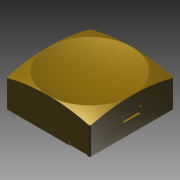
# Autodesk Inventor part: UB216SKG035D-1JBle_cap
Saved by Autodesk Inventor 2015 SP1 (Build 190203100, 203)
## iProperties
Category: Electrical
Company: Autodesk Inc.
Created: 2014-12-15
Part Number: UB216SKG035D-1JBle_cap
Catalog Web Link: http://www.nkkswitches.com/
Description: AT3074JB, AT3075B, AT3076JB-Illuminated Pushbuttons - Series UB2
Vendor: NKK Switches
Document SubType Name: Modeling
Designer: Autodesk Inc.
Manufacturer: NKKSWITCHES
Mass: 0.356668 g
Surface Area: 10.3147 cm^2
Volume: 0.356668 cm^3
Density: 1 g/cm^3
Material: Generic
Appearance: PSOLRGB-255-191-0
Title: UB216SKG035D-1JBle_cap
Author: Autodesk Inc.
Autodesk Inventor part; units mm, degrees
sketch "Sketch_2" plane through (0, 0, 0) normal (0, 0, 1) x (1, 0, 0)
  line L0 (-7.5057, 0.254) -> (7.5057, 0.254)
  line L1 (7.5057, 0.254) -> (7.5057, 6.096)
  line L2 (7.5057, 6.096) -> (-7.5057, 6.096)
  line L3 (-7.5057, 6.096) -> (-7.5057, 0.254)
  constraints: 8 end point
extrude "Extrusion1" add sketch "Sketch_2" along normal mid plane 15.0114
sketch "Sketch_20" plane through (0, 0, 0) normal (0, 1, 0) x (-1, 0, 0)
  line L0 (8.89, 8.89) -> (-8.89, 8.89)
  line L1 (-8.89, 8.89) -> (-8.89, -8.89)
  line L2 (-8.89, -8.89) -> (8.89, -8.89)
  line L3 (8.89, -8.89) -> (8.89, 8.89)
  line L4 (7.5057, -7.2517) -> (7.5057, 7.2517)
  arc A0 (7.5057, 7.2517) -> (7.2517, 7.5057) centre (7.2517, 7.2517) ccw
  line L5 (7.2517, 7.5057) -> (-7.2517, 7.5057)
  arc A1 (-7.2517, 7.5057) -> (-7.5057, 7.2517) centre (-7.2517, 7.2517) ccw
  line L6 (-7.5057, 7.2517) -> (-7.5057, -7.2517)
  arc A2 (-7.5057, -7.2517) -> (-7.2517, -7.5057) centre (-7.2517, -7.2517) ccw
  line L7 (-7.2517, -7.5057) -> (7.2517, -7.5057)
  arc A3 (7.2517, -7.5057) -> (7.5057, -7.2517) centre (7.2517, -7.2517) ccw
  constraints: 16 end point, 8 point on circle, 4 centre point
extrude "Extrusion2" cut sketch "Sketch_20" along normal blind 7.62
sketch "Sketch_9" plane through (0, 0, 0) normal (0.7071, 0, 0.7071) x (0.7071, 0, -0.7071)
  line L0 (0, 31.496) -> (0, 5.0196)
  arc A0 (-7.5057, 6.096) -> (0, 5.0196) centre (0, 31.7268) ccw
  arc A1 (-7.5057, 6.096) -> (-10.6172, 5.08) centre (0, -22.1627) ccw
  line L1 (-10.6172, 5.08) -> (-10.6172, 31.496)
  line L2 (-10.6172, 31.496) -> (0, 31.496)
  line L3 (0, 31.496) -> (0, 5.0196)
  constraints: 8 end point, 4 point on circle, 2 centre point
revolve "Revolution1" cut sketch "Sketch_9" angle 360 about axis through (0, 31.496, 0) along (0, 1, 0)
sketch "Sketch_3" plane through (0, 0, 0) normal (0, 1, 0) x (-1, 0, 0)
  line L0 (6.985, -6.985) -> (6.985, 6.985)
  line L1 (6.985, 6.985) -> (-6.985, 6.985)
  line L2 (-6.985, 6.985) -> (-6.985, -6.985)
  line L3 (-6.985, -6.985) -> (6.985, -6.985)
  constraints: 8 end point
extrude "Extrusion3" cut sketch "Sketch_3" along normal blind 4.5974
sketch "Sketch_10" plane through (0, 0, 0) normal (0, 1, 0) x (-1, 0, 0)
  line L0 (-3.81, 9.8044) -> (-6.985, 9.8044)
  line L1 (-6.985, 9.8044) -> (-6.985, 7.3787)
  line L2 (-6.985, 7.3787) -> (-3.81, 7.3787)
  line L3 (-3.81, 7.3787) -> (-3.81, 9.8044)
  constraints: 8 end point
extrude "Extrusion4" cut sketch "Sketch_10" along normal blind 1.016
sketch "Sketch_11" plane through (7.5057, 0, 0) normal (1, 0, 0) x (0, 0, -1)
  line L0 (-1.524, 2.54) -> (1.524, 2.54)
  line L1 (1.524, 2.54) -> (1.524, 3.556)
  line L2 (1.524, 3.556) -> (-1.524, 3.556)
  line L3 (-1.524, 3.556) -> (-1.524, 2.54)
  constraints: 8 end point
extrude "Extrusion5" cut sketch "Sketch_11" against normal blind 0.3387
sketch "Sketch_12" plane through (7.5057, 0, 0) normal (1, 0, 0) x (0, 0, -1)
  line L0 (-1.778, 3.556) -> (1.778, 3.556)
  line L1 (1.778, 3.556) -> (1.778, 4.826)
  line L2 (1.778, 4.826) -> (-1.778, 4.826)
  line L3 (-1.778, 4.826) -> (-1.778, 3.556)
  constraints: 8 end point
extrude "Extrusion6" cut sketch "Sketch_12" against normal blind 0.254
ref_plane "lens_to_body_XY" through (0, 0, 0) normal (0, 1, 0) x (1, 0, 0)
ref_plane "lens_to_body_YZ" through (0, 0, 0) normal (1, 0, 0) x (0, 0, -1)
ref_plane "lens_to_body_ZX" through (0, 0, 0) normal (0, 0, -1) x (0, 1, 0)
body "Solid1"
